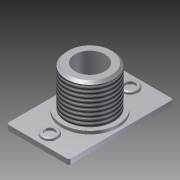
# Autodesk Inventor part: SS114-panel
Saved by Autodesk Inventor 2011 SP1 (Build 150282100, 282)
## iProperties
Created: 2013-12-24
Part Number: SS114-panel
Catalog Web Link: www.cadenas.de
Description: S Low Series-panel-Low Capacity Standard Size Toggles -panel
Vendor: NKKSWITCHES
Document SubType Name: Modeling
Designer: PARTuser1
Manufacturer: NKKSWITCHES
Density: 1 g/cm^3
Category: PARTsolutions
Company: NKKSWITCHES
Title: SS114-panel
Author: Cadenas PARTsolutions
Comments: Low Capacity Standard Size Toggles -panel
PSOL_IDENT_0: {$CADENAS_DATA\23d-libs\nkkswitches\toggle\s\parts\s_low_panel.prj},176 {VTYP=3D},{NB=SS114-panel},{
PSOL_IDENT_1: LINA=SS114-panel},{NN=S Low Series-panel},{DATE=05.04.2013 12:48:08},{GEOMDATE=05.04.2013 14:48:00},
PSOL_IDENT_2: {VERSION=},{LINEID=10},{LINESUBID=-1},{WBVAR=}  {NB=SS114-panel},{LINA=SS114-panel},{KT=DUMMY},{MDL=
PSOL_IDENT_3: S114}
CNS_NN: S Low Series-panel
CNS_NT: Low Capacity Standard Size Toggles -panel
CNS_NB: SS114-panel
CNS_NBSYN: S$MDL.-panel
CNS_LINA: SS114-panel
CNS_MDL: S114
SUPPLIER: NKKSWITCHES
ARTICLENO: SS114-panel
BOMINFO: SS114-panel
CREATOR: CADENAS GmbH
Autodesk Inventor part; units mm, degrees
sketch "Sketch_1" plane through (0, 0, 0) normal (0, 1, 0) x (-1, 0, 0)
  line L0 (7.874, -12.7) -> (7.874, 12.7)
  arc A0 (7.874, 12.7) -> (7.366, 13.208) centre (7.366, 12.7) ccw
  line L1 (7.366, 13.208) -> (-7.366, 13.208)
  arc A1 (-7.366, 13.208) -> (-7.874, 12.7) centre (-7.366, 12.7) ccw
  line L2 (-7.874, 12.7) -> (-7.874, -12.7)
  arc A2 (-7.874, -12.7) -> (-7.366, -13.208) centre (-7.366, -12.7) ccw
  line L3 (-7.366, -13.208) -> (7.366, -13.208)
  arc A3 (7.366, -13.208) -> (7.874, -12.7) centre (7.366, -12.7) ccw
  constraints: 8 end point, 8 point on circle, 4 centre point
extrude "Extrusion1" add sketch "Sketch_1" along normal blind 1.27
sketch "Sketch_4" plane through (0, 0, 0) normal (1, 0, 0) x (0, 1, 0)
  line L0 (0.762, 0) -> (11.9126, 0)
  line L1 (11.9126, -3.7592) -> (0.762, -3.7592)
  line L2 (0.762, -3.7592) -> (0.762, -7.112)
  line L3 (0.762, -7.112) -> (2.032, -7.112)
  line L4 (2.032, -7.112) -> (2.032, -6)
  line L5 (2.032, -6) -> (11.2991, -6)
  line L6 (11.2991, -6) -> (11.9126, -5.3865)
  line L7 (11.9126, -5.3865) -> (11.9126, -3.7592)
  constraints: 16 end point
revolve "Revolution1" add sketch "Sketch_4" angle 360 about axis through (0, 0.762, 0) along (0, -1, 0)
thread "Thread1" size "M12x1" class "6g" standard "ISO Metric profile" full length
sketch "Sketch_6" plane through (0, 3.81, 0) normal (0, 1, 0) x (1, 0, 0)
  line L0 (-0.508, 5.6444) -> (0.508, 5.6444)
  line L1 (0.508, 5.6444) -> (0.508, 6.4064)
  line L2 (0.508, 6.4064) -> (-0.508, 6.4064)
  line L3 (-0.508, 6.4064) -> (-0.508, 5.6444)
  constraints: 8 end point
extrude "Extrusion2" cut sketch "Sketch_6" along normal blind 25.4
sketch "Sketch_2" plane through (0, 0, -10.16) normal (0, 0, 1) x (1, 0, 0)
  line L0 (0, 1.27) -> (0, 1.905)
  line L1 (1.25, 1.27) -> (2, 1.27)
  line L2 (2, 1.27) -> (2, 1.524)
  arc A0 (2, 1.524) -> (1.619, 1.905) centre (1.619, 1.524) ccw
  line L3 (1.619, 1.905) -> (1.25, 1.905)
  line L4 (1.25, 1.905) -> (1.25, 1.27)
  constraints: 10 end point, 2 point on circle, 1 centre point
revolve "Revolution2" add sketch "Sketch_2" angle 360 about axis through (0, 1.27, -10.16) along (0, -1, 0)
sketch "Sketch_3" plane through (0, 0, 10.16) normal (0, 0, 1) x (1, 0, 0)
  line L0 (0, 1.27) -> (0, 1.905)
  line L1 (1.25, 1.27) -> (2, 1.27)
  line L2 (2, 1.27) -> (2, 1.524)
  arc A0 (2, 1.524) -> (1.619, 1.905) centre (1.619, 1.524) ccw
  line L3 (1.619, 1.905) -> (1.25, 1.905)
  line L4 (1.25, 1.905) -> (1.25, 1.27)
  constraints: 10 end point, 2 point on circle, 1 centre point
revolve "Revolution3" add sketch "Sketch_3" angle 360 about axis through (0, 1.27, 10.16) along (0, -1, 0)
ref_plane "hex_face_nut_XY" through (0, 2.032, 0) normal (0, 1, 0) x (1, 0, 0)
ref_plane "hex_face_nut_YZ" through (0, 2.032, 0) normal (1, 0, 0) x (0, 0, -1)
ref_plane "hex_face_nut_ZX" through (0, 2.032, 0) normal (0, 0, -1) x (0, 1, 0)
ref_plane "knurled_nut_XY" through (0, 4.5466, 0) normal (0, 1, 0) x (1, 0, 0)
ref_plane "knurled_nut_YZ" through (0, 4.5466, 0) normal (1, 0, 0) x (0, 0, -1)
ref_plane "knurled_nut_ZX" through (0, 4.5466, 0) normal (0, 0, -1) x (0, 1, 0)
ref_plane "lockwasher_XY" through (0, 4.0386, 0) normal (0, 1, 0) x (1, 0, 0)
ref_plane "lockwasher_YZ" through (0, 4.0386, 0) normal (1, 0, 0) x (0, 0, -1)
ref_plane "lockwasher_ZX" through (0, 4.0386, 0) normal (0, 0, -1) x (0, 1, 0)
ref_plane "panel_XY" through (0, 0, 0) normal (0, -1, 0) x (1, 0, 0)
ref_plane "panel_YZ" through (0, 0, 0) normal (1, 0, 0) x (0, 0, 1)
ref_plane "panel_ZX" through (0, 0, 0) normal (0, 0, 1) x (0, -1, 0)
ref_plane "toggle_XY" through (0, 9.4107, 0) normal (0, 1, 0) x (1, 0, 0)
ref_plane "toggle_YZ" through (0, 9.4107, 0) normal (1, 0, 0) x (0, 0, -1)
ref_plane "toggle_ZX" through (0, 9.4107, 0) normal (0, 0, -1) x (0, 1, 0)
body "Solid1"
